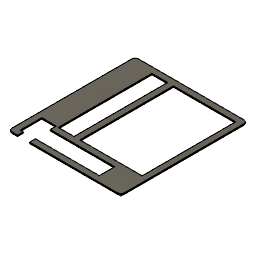
EasySplit-Left-Top (Autodesk Fusion 360 design; units mm, degrees)
part number: 2026-04-16-19-10-06-869
Autodesk Fusion 360 part; units mm, degrees
sketch "Sketch1" plane through (0, 0, 0) normal (0, 0, 1) x (1, 0, 0)
  line L0 (167.6875, -186.5) -> (-20, -186.5)
  line L1 (-10, 15) -> (157.6875, 15)
  line L2 (-20, -186.5) -> (-20, 25)
  line L3 (167.6875, 25) -> (167.6875, -186.5)
  line L4 (-10, -176.5) -> (-10, 15)
  line L5 (157.6875, 15) -> (157.6875, -176.5)
  line L6 (157.6875, -176.5) -> (-10, -176.5)
  line L7 (-20, 25) -> (167.6875, 25)
  line L8 (15, -176.5) -> (-5, -176.5)
  line L9 (-5, -176.5) -> (-5, -186.5)
  line L10 (-5, -186.5) -> (15, -186.5)
  line L11 (15, -186.5) -> (15, -176.5)
  line L12 (-10, 15) -> (18, 15)
  line L13 (18, 15) -> (18, -141)
  line L14 (18, -141) -> (-10, -141)
  line L15 (-10, -141) -> (-10, 15)
  line L16 (44, 15) -> (54, 15)
  line L17 (54, 15) -> (54, -141)
  line L18 (54, -141) -> (44, -141)
  line L19 (44, -141) -> (44, 15)
  line L20 (157.6875, -176.5) -> (121.6875, -176.5)
  line L21 (121.6875, -176.5) -> (121.6875, -141)
  line L22 (121.6875, -141) -> (157.6875, -141)
  line L23 (157.6875, -141) -> (157.6875, -176.5)
  line L24 (44, -141) -> (121.6875, -141)
  line L25 (121.6875, -141) -> (121.6875, -151)
  line L26 (121.6875, -151) -> (44, -151)
  line L27 (44, -151) -> (44, -141)
  line L28 (44, -151) -> (18, -151)
  line L29 (18, -151) -> (18, -141)
  line L30 (18, -141) -> (44, -141)
  line L31 (44, -141) -> (44, -151)
  line L32 (14, -141) -> (18, -141)
  line L33 (18, -141) -> (18, -151)
  line L34 (18, -151) -> (14, -151)
  line L35 (14, -151) -> (14, -141)
  dimension "d3" = 167.6875
  dimension "d4" = 191.5
  dimension "d5" = 187.6875
  dimension "d6" = 211.5
  dimension "d7" = 10
  dimension "d8" = 10
  dimension "d19" = 20
  dimension "d20" = 15
  dimension "d21" = 28
  dimension "d22" = 156
  dimension "d23" = 10
  dimension "d24" = 156
  dimension "d25" = 26
  dimension "d26" = 36
  dimension "d27" = 35.5
  dimension "d28" = 10
  constraint horizontal L1
  constraint vertical L5
  constraint horizontal L6
  constraint vertical L4
  constraint horizontal L7
  constraint vertical L3
  constraint horizontal L0
  constraint vertical L2
  constraint horizontal L8
  constraint vertical L9
  constraint horizontal L10
  constraint vertical L11
  constraint coincident L6 L8.start
  constraint horizontal L12
  constraint vertical L13
  constraint horizontal L14
  constraint vertical L15
  constraint horizontal L16
  constraint vertical L17
  constraint horizontal L18
  constraint vertical L19
  constraint coincident L1 L16.start
  constraint horizontal L20
  constraint vertical L21
  constraint horizontal L22
  constraint vertical L23
  constraint horizontal L24
  constraint vertical L25
  constraint horizontal L26
  constraint vertical L27
  constraint coincident L21 L25.end
  constraint horizontal L28
  constraint vertical L29
  constraint horizontal L30
  constraint vertical L31
  constraint horizontal L32
  constraint vertical L33
  constraint horizontal L34
  constraint vertical L35
  constraint coincident L14 L32.start
  measures "d3" distance of L1.start L1.end
  measures "d4" distance of L1.start L4.start
  measures "d5" distance of L2.end L3.start
  measures "d6" distance of L2.end L0.end
  measures "d7" distance of L1 L7
  measures "d8" distance of L2 L4
  measures "d19" distance of L8.start L8.end
  measures "d20" distance of L2 L9
  measures "d21" distance of L1.start L12.end
  measures "d22" distance of L1.start L14.end
  measures "d23" distance of L16.start L16.end
  measures "d24" distance of L16.start L18.end
  measures "d25" distance of L13 L19
  measures "d26" distance of L5.end L20.end
  measures "d27" distance of L5.end L22.end
  measures "d28" distance of L18.end L26.end
extrude "Extrude1" add sketch "Sketch1" along normal blind 2 contours L0 L1 L2 L3 L4 L5 L6 L7 L9 L11 L12 L15 L16 L20 L23 | L5 L6 L20 L21 L22 L23 L25 | L18 L21 L24 L25 L26 L27 L31 | L1 L4 L12 L13 L14 L15 L32 | L27 L28 L29 L30 L31 L33 | L14 L29 L32 L33 L34 L35 | L1 L16 L17 L18 L19 L24
fillet "Fillet1" radius 6 1 edges at (167.6875, -186.5, 1)
fillet "Fillet2" radius 6 1 edges at (167.6875, 25, 1)
fillet "Fillet3" radius 6 1 edges at (-20, 25, 1)
fillet "Fillet4" radius 6 1 edges at (-20, -186.5, 1)
sketch "Sketch2" plane through (0, 0, 2) normal (0, 0, 1) x (-1, 0, 0)
  arc A0 (20, 180.5) -> (14, 186.5) centre (14, 180.5) ccw
  line L0 (14, 186.5) -> (5, 186.5)
  line L1 (5, 186.5) -> (5, 176.5)
  line L2 (5, 176.5) -> (10, 176.5)
  line L3 (10, 176.5) -> (10, 141)
  line L4 (10, 141) -> (-14, 141)
  line L5 (-14, 141) -> (-14, 151)
  line L6 (-14, 151) -> (-121.6875, 151)
  line L7 (-121.6875, 151) -> (-121.6875, 176.5)
  line L8 (-121.6875, 176.5) -> (-15, 176.5)
  line L9 (-15, 176.5) -> (-15, 186.5)
  line L10 (-15, 186.5) -> (-161.6875, 186.5)
  arc A1 (-161.6875, 186.5) -> (-167.6875, 180.5) centre (-161.6875, 180.5) ccw
  line L11 (-167.6875, 180.5) -> (-167.6875, -19)
  arc A2 (-167.6875, -19) -> (-161.6875, -25) centre (-161.6875, -19) ccw
  line L12 (-161.6875, -25) -> (14, -25)
  arc A3 (14, -25) -> (20, -19) centre (14, -19) ccw
  line L13 (20, -19) -> (20, 180.5)
  line L14 (-18, 141) -> (-18, -15)
  line L15 (-18, -15) -> (-44, -15)
  line L16 (-44, -15) -> (-44, 141)
  line L17 (-44, 141) -> (-18, 141)
  line L18 (-54, -15) -> (-157.6875, -15)
  line L19 (-157.6875, -15) -> (-157.6875, 141)
  line L20 (-157.6875, 141) -> (-54, 141)
  line L21 (-54, 141) -> (-54, -15)
  circle A4 centre (14, -19) radius 2.1
  circle A5 centre (-161.6875, -19) radius 2.1
  circle A6 centre (-161.6875, 180.5) radius 2.1
  circle A7 centre (14, 180.5) radius 2.1
  dimension "d29" = 4.2
  dimension "d30" = 4.2
  dimension "d31" = 4.2
  dimension "d32" = 4.2
  dimension "d33" = 6
  dimension "d34" = 6
  dimension "d35" = 6
  dimension "d36" = 6
  dimension "d37" = 6
  dimension "d38" = 6
  dimension "d39" = 6
  dimension "d40" = 6
  measures "d29" diameter of A4
  measures "d30" diameter of A5
  measures "d31" diameter of A6
  measures "d32" diameter of A7
  measures "d33" distance of L0 A0.centre
  measures "d34" distance of L13 A0.centre
  measures "d35" distance of L12 A3.centre
  measures "d36" distance of L13 A3.centre
  measures "d37" distance of L12 A2.centre
  measures "d38" distance of L11 A2.centre
  measures "d39" distance of L10 A1.centre
  measures "d40" distance of L11 A1.centre
extrude "Extrude2" add sketch "Sketch2" against normal blind 6 contours A4 | A5 | A6 | A7
